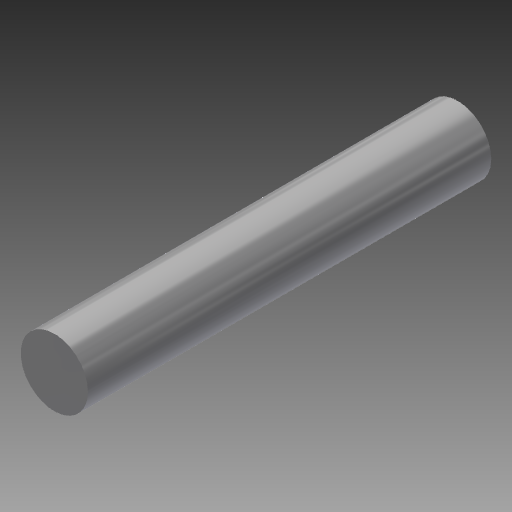
# Autodesk Inventor part: Flache Riemenscheibe1
Saved by Autodesk Inventor 2019.1 (Build 231200000, 200)
## iProperties
Created: 2018-11-01
Part Number: Flache Riemenscheibe1
Material: Steel
Document SubType Name: Modeling
Designer: JochenAlt
Density: 7.85 g/cm^3
Appearance: Steel
CustomPartVersion: 1
Author: JochenAlt
Autodesk Inventor part; units mm, degrees
ref_plane "YZ Plane" through (0, 0, 0) normal (1, 0, 0) x (0, 1, 0)
ref_plane "XZ Plane" through (0, 0, 0) normal (0, 1, 0) x (-1, 0, 0)
ref_plane "XY Plane" through (0, 0, 0) normal (0, 0, 1) x (1, 0, 0)
sketch "Hauptskizze" plane through (0, 0, 0) normal (0, 0, 1) x (1, 0, 0)
  circle A0 centre (0, 0) radius 1
  dimension "d0" = 2
  constraints: 1 centre point, 1 coincident
  measures "d0" diameter of A0
extrude "Riemenscheibe" add sketch "Hauptskizze" along normal mid plane 12
equation "\"d0\" = da_D"
equation "\"d1\" = da_B"
equation "\"da_D\" = 2"
equation "\"da_B\" = 12"
body "Solid1"
